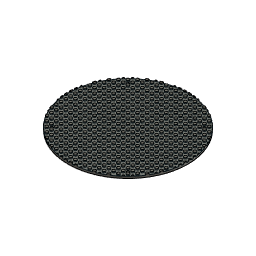
cartAssembly v25 (Autodesk Fusion 360 archive; units mm, degrees)
design "flat legosetup"
Autodesk Fusion 360 part; units mm, degrees
sketch "Sketch1" plane through (0, 0, 0) normal (0, 1, 0) x (1, 0, 0)
  line L0 (-119.9, -119.9) -> (119.9, -119.9)
  line L1 (119.9, -119.9) -> (119.9, 119.9)
  line L2 (119.9, 119.9) -> (-119.9, 119.9)
  line L3 (-119.9, 119.9) -> (-119.9, -119.9)
  line L4 (-119.9, -119.9) -> (119.9, 119.9) construction
  line L5 (119.9, -119.9) -> (-119.9, 119.9) construction
  dimension "d5" = 239.8
  dimension "d6" = 239.8
  constraint horizontal L0
  constraint perpendicular L0 L1
  constraint parallel L0 L2
  constraint parallel L1 L3
  constraint coincident L4 origin
  constraint coincident L5 origin
  measures "d5" distance of L1.end L2.end
  measures "d6" distance of L0.start L2.end
extrude "Extrude1" add sketch "Sketch1" along normal blind 3.2 makes body 1
sketch "Sketch2" plane through (0, 3.2, 0) normal (0, 1, 0) x (-1, 0, 0)
  line L0 (119.9, -119.9) -> (119.9, 119.9)
  line L1 (119.9, 119.9) -> (-119.9, 119.9)
  line L2 (-119.9, 119.9) -> (-119.9, -119.9)
  line L3 (-119.9, -119.9) -> (119.9, -119.9)
  circle A0 centre (116, -116) radius 2.4
  dimension "d9" = 4.8
  dimension "d10" = 3.9
  dimension "d11" = 3.9
  measures "d9" diameter of A0
  measures "d10" distance of L3 A0.centre
  measures "d11" distance of L0 A0.centre
extrude "Extrude2" add sketch "Sketch2" along normal blind 1.8 contours A0 bodies 1
pattern_linear "R-Pattern1" count 30 spacing 8 along (1, 0, 0) count 30 spacing 8 along (0, 0, 1) of "Extrude2"
cylinder "CylinderPrimitive1" add diameter 200 height 20 placed x (1, 0, 0) y (0, 0, -1) z (0, 1, 0) at (0, 3.2, 0) separate body makes body 2
move_body "Move1" bodies 2 to x (1, 0, 0) y (0, 1, 0) z (0, 0, 1) at (0, -10, 0)
combine "Combine1" operation intersect target body 1 tool bodies 2
sketch "Sketch4" plane through (0, 3.2, 0) normal (0, 1, 0) x (-1, 0, 0)
  arc A0 (-14.1771, 98.9899) -> (-18.2934, 98.3125) centre (0, 0) ccw
  arc A1 (-20.9263, 97.7859) -> (-18.2934, 98.3125) centre (-20, 100) ccw
  arc A2 (-20.9263, 97.7859) -> (-34.4887, 93.8644) centre (0, 0) ccw
  arc A3 (-38.3753, 92.3436) -> (-34.4887, 93.8644) centre (-36, 92) ccw
  arc A4 (-38.3753, 92.3436) -> (-41.9306, 90.7845) centre (0, 0) ccw
  arc A5 (-44.3528, 89.6261) -> (-41.9306, 90.7845) centre (-44, 92) ccw
  arc A6 (-44.3528, 89.6261) -> (-50.8497, 86.1064) centre (0, 0) ccw
  arc A7 (-54.3983, 83.9096) -> (-50.8497, 86.1064) centre (-52, 84) ccw
  arc A8 (-54.3983, 83.9096) -> (-65.673, 75.4126) centre (0, 0) ccw
  arc A9 (-67.674, 73.6222) -> (-65.673, 75.4126) centre (-68, 76) ccw
  arc A10 (-67.674, 73.6222) -> (-73.6222, 67.674) centre (0, 0) ccw
  arc A11 (-75.4126, 65.673) -> (-73.6222, 67.674) centre (-76, 68) ccw
  arc A12 (-75.4126, 65.673) -> (-83.9096, 54.3983) centre (0, 0) ccw
  arc A13 (-86.1064, 50.8497) -> (-83.9096, 54.3983) centre (-84, 52) ccw
  arc A14 (-86.1064, 50.8497) -> (-89.6261, 44.3528) centre (0, 0) ccw
  arc A15 (-90.7845, 41.9306) -> (-89.6261, 44.3528) centre (-92, 44) ccw
  arc A16 (-90.7845, 41.9306) -> (-92.3436, 38.3753) centre (0, 0) ccw
  arc A17 (-93.8644, 34.4887) -> (-92.3436, 38.3753) centre (-92, 36) ccw
  arc A18 (-93.8644, 34.4887) -> (-97.7859, 20.9263) centre (0, 0) ccw
  arc A19 (-98.3125, 18.2934) -> (-97.7859, 20.9263) centre (-100, 20) ccw
  arc A20 (-98.3125, 18.2934) -> (-98.9899, 14.1771) centre (0, 0) ccw
  arc A21 (-99.5337, 9.6457) -> (-98.9899, 14.1771) centre (-100, 12) ccw
  arc A22 (-99.5337, 9.6457) -> (-99.7955, 6.3913) centre (0, 0) ccw
  arc A23 (-99.9872, 1.6) -> (-99.7955, 6.3913) centre (-100, 4) ccw
  arc A24 (-99.9872, 1.6) -> (-99.9872, -1.6) centre (0, 0) ccw
  arc A25 (-99.7955, -6.3913) -> (-99.9872, -1.6) centre (-100, -4) ccw
  arc A26 (-99.7955, -6.3913) -> (-99.5337, -9.6457) centre (0, 0) ccw
  arc A27 (-98.9899, -14.1771) -> (-99.5337, -9.6457) centre (-100, -12) ccw
  arc A28 (-98.9899, -14.1771) -> (-98.3125, -18.2934) centre (0, 0) ccw
  arc A29 (-97.7859, -20.9263) -> (-98.3125, -18.2934) centre (-100, -20) ccw
  arc A30 (-97.7859, -20.9263) -> (-93.8644, -34.4887) centre (0, 0) ccw
  arc A31 (-92.3436, -38.3753) -> (-93.8644, -34.4887) centre (-92, -36) ccw
  arc A32 (-92.3436, -38.3753) -> (-90.7845, -41.9306) centre (0, 0) ccw
  arc A33 (-89.6261, -44.3528) -> (-90.7845, -41.9306) centre (-92, -44) ccw
  arc A34 (-89.6261, -44.3528) -> (-86.1064, -50.8497) centre (0, 0) ccw
  arc A35 (-83.9096, -54.3983) -> (-86.1064, -50.8497) centre (-84, -52) ccw
  arc A36 (-83.9096, -54.3983) -> (-75.4126, -65.673) centre (0, 0) ccw
  arc A37 (-73.6222, -67.674) -> (-75.4126, -65.673) centre (-76, -68) ccw
  arc A38 (-73.6222, -67.674) -> (-67.674, -73.6222) centre (0, 0) ccw
  arc A39 (-65.673, -75.4126) -> (-67.674, -73.6222) centre (-68, -76) ccw
  arc A40 (-65.673, -75.4126) -> (-54.3983, -83.9096) centre (0, 0) ccw
  arc A41 (-50.8497, -86.1064) -> (-54.3983, -83.9096) centre (-52, -84) ccw
  arc A42 (-50.8497, -86.1064) -> (-44.3528, -89.6261) centre (0, 0) ccw
  arc A43 (-41.9306, -90.7845) -> (-44.3528, -89.6261) centre (-44, -92) ccw
  arc A44 (-41.9306, -90.7845) -> (-38.3753, -92.3436) centre (0, 0) ccw
  arc A45 (-34.4887, -93.8644) -> (-38.3753, -92.3436) centre (-36, -92) ccw
  arc A46 (-34.4887, -93.8644) -> (-20.9263, -97.7859) centre (0, 0) ccw
  arc A47 (-18.2934, -98.3125) -> (-20.9263, -97.7859) centre (-20, -100) ccw
  arc A48 (-18.2934, -98.3125) -> (-14.1771, -98.9899) centre (0, 0) ccw
  arc A49 (-9.6457, -99.5337) -> (-14.1771, -98.9899) centre (-12, -100) ccw
  arc A50 (-9.6457, -99.5337) -> (-6.3913, -99.7955) centre (0, 0) ccw
  arc A51 (-1.6, -99.9872) -> (-6.3913, -99.7955) centre (-4, -100) ccw
  arc A52 (-1.6, -99.9872) -> (1.6, -99.9872) centre (0, 0) ccw
  arc A53 (6.3913, -99.7955) -> (1.6, -99.9872) centre (4, -100) ccw
  arc A54 (6.3913, -99.7955) -> (9.6457, -99.5337) centre (0, 0) ccw
  arc A55 (14.1771, -98.9899) -> (9.6457, -99.5337) centre (12, -100) ccw
  arc A56 (14.1771, -98.9899) -> (18.2934, -98.3125) centre (0, 0) ccw
  arc A57 (20.9263, -97.7859) -> (18.2934, -98.3125) centre (20, -100) ccw
  arc A58 (20.9263, -97.7859) -> (34.4887, -93.8644) centre (0, 0) ccw
  arc A59 (38.3753, -92.3436) -> (34.4887, -93.8644) centre (36, -92) ccw
  arc A60 (38.3753, -92.3436) -> (41.9306, -90.7845) centre (0, 0) ccw
  arc A61 (44.3528, -89.6261) -> (41.9306, -90.7845) centre (44, -92) ccw
  arc A62 (44.3528, -89.6261) -> (50.8497, -86.1064) centre (0, 0) ccw
  arc A63 (54.3983, -83.9096) -> (50.8497, -86.1064) centre (52, -84) ccw
  arc A64 (54.3983, -83.9096) -> (65.673, -75.4126) centre (0, 0) ccw
  arc A65 (67.674, -73.6222) -> (65.673, -75.4126) centre (68, -76) ccw
  arc A66 (67.674, -73.6222) -> (73.6222, -67.674) centre (0, 0) ccw
  arc A67 (75.4126, -65.673) -> (73.6222, -67.674) centre (76, -68) ccw
  arc A68 (75.4126, -65.673) -> (83.9096, -54.3983) centre (0, 0) ccw
  arc A69 (86.1064, -50.8497) -> (83.9096, -54.3983) centre (84, -52) ccw
  arc A70 (86.1064, -50.8497) -> (89.6261, -44.3528) centre (0, 0) ccw
  arc A71 (90.7845, -41.9306) -> (89.6261, -44.3528) centre (92, -44) ccw
  arc A72 (90.7845, -41.9306) -> (92.3436, -38.3753) centre (0, 0) ccw
  arc A73 (93.8644, -34.4887) -> (92.3436, -38.3753) centre (92, -36) ccw
  arc A74 (93.8644, -34.4887) -> (97.7859, -20.9263) centre (0, 0) ccw
  arc A75 (98.3125, -18.2934) -> (97.7859, -20.9263) centre (100, -20) ccw
  arc A76 (98.3125, -18.2934) -> (98.9899, -14.1771) centre (0, 0) ccw
  arc A77 (99.5337, -9.6457) -> (98.9899, -14.1771) centre (100, -12) ccw
  arc A78 (99.5337, -9.6457) -> (99.7955, -6.3913) centre (0, 0) ccw
  arc A79 (99.9872, -1.6) -> (99.7955, -6.3913) centre (100, -4) ccw
  arc A80 (99.9872, -1.6) -> (99.9872, 1.6) centre (0, 0) ccw
  arc A81 (99.7955, 6.3913) -> (99.9872, 1.6) centre (100, 4) ccw
  arc A82 (99.7955, 6.3913) -> (99.5337, 9.6457) centre (0, 0) ccw
  arc A83 (98.9899, 14.1771) -> (99.5337, 9.6457) centre (100, 12) ccw
  arc A84 (98.9899, 14.1771) -> (98.3125, 18.2934) centre (0, 0) ccw
  arc A85 (97.7859, 20.9263) -> (98.3125, 18.2934) centre (100, 20) ccw
  arc A86 (97.7859, 20.9263) -> (93.8644, 34.4887) centre (0, 0) ccw
  arc A87 (92.3436, 38.3753) -> (93.8644, 34.4887) centre (92, 36) ccw
  arc A88 (92.3436, 38.3753) -> (90.7845, 41.9306) centre (0, 0) ccw
  arc A89 (89.6261, 44.3528) -> (90.7845, 41.9306) centre (92, 44) ccw
  arc A90 (89.6261, 44.3528) -> (86.1064, 50.8497) centre (0, 0) ccw
  arc A91 (83.9096, 54.3983) -> (86.1064, 50.8497) centre (84, 52) ccw
  arc A92 (83.9096, 54.3983) -> (75.4126, 65.673) centre (0, 0) ccw
  arc A93 (73.6222, 67.674) -> (75.4126, 65.673) centre (76, 68) ccw
  arc A94 (73.6222, 67.674) -> (67.674, 73.6222) centre (0, 0) ccw
  arc A95 (65.673, 75.4126) -> (67.674, 73.6222) centre (68, 76) ccw
  arc A96 (65.673, 75.4126) -> (54.3983, 83.9096) centre (0, 0) ccw
  arc A97 (50.8497, 86.1064) -> (54.3983, 83.9096) centre (52, 84) ccw
  arc A98 (50.8497, 86.1064) -> (44.3528, 89.6261) centre (0, 0) ccw
  arc A99 (41.9306, 90.7845) -> (44.3528, 89.6261) centre (44, 92) ccw
  arc A100 (41.9306, 90.7845) -> (38.3753, 92.3436) centre (0, 0) ccw
  arc A101 (34.4887, 93.8644) -> (38.3753, 92.3436) centre (36, 92) ccw
  arc A102 (34.4887, 93.8644) -> (20.9263, 97.7859) centre (0, 0) ccw
  arc A103 (18.2934, 98.3125) -> (20.9263, 97.7859) centre (20, 100) ccw
  arc A104 (18.2934, 98.3125) -> (14.1771, 98.9899) centre (0, 0) ccw
  arc A105 (9.6457, 99.5337) -> (14.1771, 98.9899) centre (12, 100) ccw
  arc A106 (9.6457, 99.5337) -> (6.3913, 99.7955) centre (0, 0) ccw
  arc A107 (1.6, 99.9872) -> (6.3913, 99.7955) centre (4, 100) ccw
  arc A108 (1.6, 99.9872) -> (-1.6, 99.9872) centre (0, 0) ccw
  arc A109 (-6.3913, 99.7955) -> (-1.6, 99.9872) centre (-4, 100) ccw
  arc A110 (-6.3913, 99.7955) -> (-9.6457, 99.5337) centre (0, 0) ccw
  arc A111 (-14.1771, 98.9899) -> (-9.6457, 99.5337) centre (-12, 100) ccw
  circle A112 centre (-28, 92) radius 2.4
  circle A113 centre (-20, 92) radius 2.4
  circle A114 centre (-12, 92) radius 2.4
  circle A115 centre (-4, 92) radius 2.4
  circle A116 centre (4, 92) radius 2.4
  circle A117 centre (12, 92) radius 2.4
  circle A118 centre (20, 92) radius 2.4
  circle A119 centre (28, 92) radius 2.4
  circle A120 centre (-44, 84) radius 2.4
  circle A121 centre (-36, 84) radius 2.4
  circle A122 centre (-28, 84) radius 2.4
  circle A123 centre (-20, 84) radius 2.4
  circle A124 centre (-12, 84) radius 2.4
  circle A125 centre (-4, 84) radius 2.4
  circle A126 centre (4, 84) radius 2.4
  circle A127 centre (12, 84) radius 2.4
  circle A128 centre (20, 84) radius 2.4
  circle A129 centre (28, 84) radius 2.4
  circle A130 centre (36, 84) radius 2.4
  circle A131 centre (44, 84) radius 2.4
  circle A132 centre (-60, 76) radius 2.4
  circle A133 centre (-52, 76) radius 2.4
  circle A134 centre (-44, 76) radius 2.4
  circle A135 centre (-36, 76) radius 2.4
  circle A136 centre (-28, 76) radius 2.4
  circle A137 centre (-20, 76) radius 2.4
  circle A138 centre (-12, 76) radius 2.4
  circle A139 centre (-4, 76) radius 2.4
  circle A140 centre (4, 76) radius 2.4
  circle A141 centre (12, 76) radius 2.4
  circle A142 centre (20, 76) radius 2.4
  circle A143 centre (28, 76) radius 2.4
  circle A144 centre (36, 76) radius 2.4
  circle A145 centre (44, 76) radius 2.4
  circle A146 centre (52, 76) radius 2.4
  circle A147 centre (60, 76) radius 2.4
  circle A148 centre (-68, 68) radius 2.4
  circle A149 centre (-60, 68) radius 2.4
  circle A150 centre (-52, 68) radius 2.4
  circle A151 centre (-44, 68) radius 2.4
  circle A152 centre (-36, 68) radius 2.4
  circle A153 centre (-28, 68) radius 2.4
  circle A154 centre (-20, 68) radius 2.4
  circle A155 centre (-12, 68) radius 2.4
  circle A156 centre (-4, 68) radius 2.4
  circle A157 centre (4, 68) radius 2.4
  circle A158 centre (12, 68) radius 2.4
  circle A159 centre (20, 68) radius 2.4
  circle A160 centre (28, 68) radius 2.4
  circle A161 centre (36, 68) radius 2.4
  circle A162 centre (44, 68) radius 2.4
  circle A163 centre (52, 68) radius 2.4
  circle A164 centre (60, 68) radius 2.4
  circle A165 centre (68, 68) radius 2.4
  circle A166 centre (-76, 60) radius 2.4
  circle A167 centre (-68, 60) radius 2.4
  circle A168 centre (-60, 60) radius 2.4
  circle A169 centre (-52, 60) radius 2.4
  circle A170 centre (-44, 60) radius 2.4
  circle A171 centre (-36, 60) radius 2.4
  circle A172 centre (-28, 60) radius 2.4
  circle A173 centre (-20, 60) radius 2.4
  circle A174 centre (-12, 60) radius 2.4
  circle A175 centre (-4, 60) radius 2.4
  circle A176 centre (4, 60) radius 2.4
  circle A177 centre (12, 60) radius 2.4
  circle A178 centre (20, 60) radius 2.4
  circle A179 centre (28, 60) radius 2.4
  circle A180 centre (36, 60) radius 2.4
  circle A181 centre (44, 60) radius 2.4
  circle A182 centre (52, 60) radius 2.4
  circle A183 centre (60, 60) radius 2.4
  circle A184 centre (68, 60) radius 2.4
  circle A185 centre (76, 60) radius 2.4
  circle A186 centre (-76, 52) radius 2.4
  circle A187 centre (-68, 52) radius 2.4
  circle A188 centre (-60, 52) radius 2.4
  circle A189 centre (-52, 52) radius 2.4
  circle A190 centre (-44, 52) radius 2.4
  circle A191 centre (-36, 52) radius 2.4
  circle A192 centre (-28, 52) radius 2.4
  circle A193 centre (-20, 52) radius 2.4
  circle A194 centre (-12, 52) radius 2.4
  circle A195 centre (-4, 52) radius 2.4
  circle A196 centre (4, 52) radius 2.4
  circle A197 centre (12, 52) radius 2.4
  circle A198 centre (20, 52) radius 2.4
  circle A199 centre (28, 52) radius 2.4
  circle A200 centre (36, 52) radius 2.4
  circle A201 centre (44, 52) radius 2.4
  circle A202 centre (52, 52) radius 2.4
  circle A203 centre (60, 52) radius 2.4
  circle A204 centre (68, 52) radius 2.4
  circle A205 centre (76, 52) radius 2.4
  circle A206 centre (-84, 44) radius 2.4
  circle A207 centre (-76, 44) radius 2.4
  circle A208 centre (-68, 44) radius 2.4
  circle A209 centre (-60, 44) radius 2.4
  circle A210 centre (-52, 44) radius 2.4
  circle A211 centre (-44, 44) radius 2.4
  circle A212 centre (-36, 44) radius 2.4
  circle A213 centre (-28, 44) radius 2.4
  circle A214 centre (-20, 44) radius 2.4
  circle A215 centre (-12, 44) radius 2.4
  circle A216 centre (-4, 44) radius 2.4
  circle A217 centre (4, 44) radius 2.4
  circle A218 centre (12, 44) radius 2.4
  circle A219 centre (20, 44) radius 2.4
  circle A220 centre (28, 44) radius 2.4
  circle A221 centre (36, 44) radius 2.4
  circle A222 centre (44, 44) radius 2.4
  circle A223 centre (52, 44) radius 2.4
  circle A224 centre (60, 44) radius 2.4
  circle A225 centre (68, 44) radius 2.4
  circle A226 centre (76, 44) radius 2.4
  circle A227 centre (84, 44) radius 2.4
  circle A228 centre (-84, 36) radius 2.4
  circle A229 centre (-76, 36) radius 2.4
  circle A230 centre (-68, 36) radius 2.4
  circle A231 centre (-60, 36) radius 2.4
  circle A232 centre (-52, 36) radius 2.4
  circle A233 centre (-44, 36) radius 2.4
  circle A234 centre (-36, 36) radius 2.4
  circle A235 centre (-28, 36) radius 2.4
  circle A236 centre (-20, 36) radius 2.4
  circle A237 centre (-12, 36) radius 2.4
  circle A238 centre (-4, 36) radius 2.4
  circle A239 centre (4, 36) radius 2.4
  circle A240 centre (12, 36) radius 2.4
  circle A241 centre (20, 36) radius 2.4
  circle A242 centre (28, 36) radius 2.4
  circle A243 centre (36, 36) radius 2.4
  circle A244 centre (44, 36) radius 2.4
  circle A245 centre (52, 36) radius 2.4
  circle A246 centre (60, 36) radius 2.4
  circle A247 centre (68, 36) radius 2.4
  circle A248 centre (76, 36) radius 2.4
  circle A249 centre (84, 36) radius 2.4
  circle A250 centre (-92, 28) radius 2.4
  circle A251 centre (-84, 28) radius 2.4
  circle A252 centre (-76, 28) radius 2.4
  circle A253 centre (-68, 28) radius 2.4
  circle A254 centre (-60, 28) radius 2.4
  circle A255 centre (-52, 28) radius 2.4
  circle A256 centre (-44, 28) radius 2.4
  circle A257 centre (-36, 28) radius 2.4
  circle A258 centre (-28, 28) radius 2.4
  circle A259 centre (-20, 28) radius 2.4
  circle A260 centre (-12, 28) radius 2.4
  circle A261 centre (-4, 28) radius 2.4
  circle A262 centre (4, 28) radius 2.4
  circle A263 centre (12, 28) radius 2.4
  circle A264 centre (20, 28) radius 2.4
  circle A265 centre (28, 28) radius 2.4
  circle A266 centre (36, 28) radius 2.4
  circle A267 centre (44, 28) radius 2.4
  circle A268 centre (52, 28) radius 2.4
  circle A269 centre (60, 28) radius 2.4
  circle A270 centre (68, 28) radius 2.4
  circle A271 centre (76, 28) radius 2.4
  circle A272 centre (84, 28) radius 2.4
  circle A273 centre (92, 28) radius 2.4
  circle A274 centre (-92, 20) radius 2.4
  circle A275 centre (-84, 20) radius 2.4
  circle A276 centre (-76, 20) radius 2.4
  circle A277 centre (-68, 20) radius 2.4
  circle A278 centre (-60, 20) radius 2.4
  circle A279 centre (-52, 20) radius 2.4
  circle A280 centre (-44, 20) radius 2.4
  circle A281 centre (-36, 20) radius 2.4
  circle A282 centre (-28, 20) radius 2.4
  circle A283 centre (-20, 20) radius 2.4
  circle A284 centre (-12, 20) radius 2.4
  circle A285 centre (-4, 20) radius 2.4
  circle A286 centre (4, 20) radius 2.4
  circle A287 centre (12, 20) radius 2.4
  circle A288 centre (20, 20) radius 2.4
  circle A289 centre (28, 20) radius 2.4
  circle A290 centre (36, 20) radius 2.4
  circle A291 centre (44, 20) radius 2.4
  circle A292 centre (52, 20) radius 2.4
  circle A293 centre (60, 20) radius 2.4
  circle A294 centre (68, 20) radius 2.4
  circle A295 centre (76, 20) radius 2.4
  circle A296 centre (84, 20) radius 2.4
  circle A297 centre (92, 20) radius 2.4
  circle A298 centre (-92, 12) radius 2.4
  circle A299 centre (-84, 12) radius 2.4
  circle A300 centre (-76, 12) radius 2.4
  circle A301 centre (-68, 12) radius 2.4
  circle A302 centre (-60, 12) radius 2.4
  circle A303 centre (-52, 12) radius 2.4
  circle A304 centre (-44, 12) radius 2.4
  circle A305 centre (-36, 12) radius 2.4
  circle A306 centre (-28, 12) radius 2.4
  circle A307 centre (-20, 12) radius 2.4
  circle A308 centre (-12, 12) radius 2.4
  circle A309 centre (-4, 12) radius 2.4
  circle A310 centre (4, 12) radius 2.4
  circle A311 centre (12, 12) radius 2.4
  circle A312 centre (20, 12) radius 2.4
  circle A313 centre (28, 12) radius 2.4
  circle A314 centre (36, 12) radius 2.4
  circle A315 centre (44, 12) radius 2.4
  circle A316 centre (52, 12) radius 2.4
  circle A317 centre (60, 12) radius 2.4
  circle A318 centre (68, 12) radius 2.4
  circle A319 centre (76, 12) radius 2.4
  circle A320 centre (84, 12) radius 2.4
  circle A321 centre (92, 12) radius 2.4
  circle A322 centre (-92, 4) radius 2.4
  circle A323 centre (-84, 4) radius 2.4
  circle A324 centre (-76, 4) radius 2.4
  circle A325 centre (-68, 4) radius 2.4
  circle A326 centre (-60, 4) radius 2.4
  circle A327 centre (-52, 4) radius 2.4
  circle A328 centre (-44, 4) radius 2.4
  circle A329 centre (-36, 4) radius 2.4
  circle A330 centre (-28, 4) radius 2.4
  circle A331 centre (-20, 4) radius 2.4
  circle A332 centre (-12, 4) radius 2.4
  circle A333 centre (-4, 4) radius 2.4
  circle A334 centre (4, 4) radius 2.4
  circle A335 centre (12, 4) radius 2.4
  circle A336 centre (20, 4) radius 2.4
  circle A337 centre (28, 4) radius 2.4
  circle A338 centre (36, 4) radius 2.4
  circle A339 centre (44, 4) radius 2.4
  circle A340 centre (52, 4) radius 2.4
  circle A341 centre (60, 4) radius 2.4
  circle A342 centre (68, 4) radius 2.4
  circle A343 centre (76, 4) radius 2.4
  circle A344 centre (84, 4) radius 2.4
  circle A345 centre (92, 4) radius 2.4
  circle A346 centre (-92, -4) radius 2.4
  circle A347 centre (-84, -4) radius 2.4
  circle A348 centre (-76, -4) radius 2.4
  circle A349 centre (-68, -4) radius 2.4
  circle A350 centre (-60, -4) radius 2.4
  circle A351 centre (-52, -4) radius 2.4
  circle A352 centre (-44, -4) radius 2.4
  circle A353 centre (-36, -4) radius 2.4
  circle A354 centre (-28, -4) radius 2.4
  circle A355 centre (-20, -4) radius 2.4
  circle A356 centre (-12, -4) radius 2.4
  circle A357 centre (-4, -4) radius 2.4
  circle A358 centre (4, -4) radius 2.4
  circle A359 centre (12, -4) radius 2.4
  circle A360 centre (20, -4) radius 2.4
  circle A361 centre (28, -4) radius 2.4
  circle A362 centre (36, -4) radius 2.4
  circle A363 centre (44, -4) radius 2.4
  circle A364 centre (52, -4) radius 2.4
  circle A365 centre (60, -4) radius 2.4
  circle A366 centre (68, -4) radius 2.4
  circle A367 centre (76, -4) radius 2.4
  circle A368 centre (84, -4) radius 2.4
  circle A369 centre (92, -4) radius 2.4
  circle A370 centre (-92, -12) radius 2.4
  circle A371 centre (-84, -12) radius 2.4
  circle A372 centre (-76, -12) radius 2.4
  circle A373 centre (-68, -12) radius 2.4
  circle A374 centre (-60, -12) radius 2.4
  circle A375 centre (-52, -12) radius 2.4
  circle A376 centre (-44, -12) radius 2.4
  circle A377 centre (-36, -12) radius 2.4
  circle A378 centre (-28, -12) radius 2.4
  circle A379 centre (-20, -12) radius 2.4
  circle A380 centre (-12, -12) radius 2.4
  circle A381 centre (-4, -12) radius 2.4
  circle A382 centre (4, -12) radius 2.4
  circle A383 centre (12, -12) radius 2.4
  circle A384 centre (20, -12) radius 2.4
  circle A385 centre (28, -12) radius 2.4
  circle A386 centre (36, -12) radius 2.4
  circle A387 centre (44, -12) radius 2.4
  circle A388 centre (52, -12) radius 2.4
  circle A389 centre (60, -12) radius 2.4
  circle A390 centre (68, -12) radius 2.4
  circle A391 centre (76, -12) radius 2.4
  circle A392 centre (84, -12) radius 2.4
  circle A393 centre (92, -12) radius 2.4
  circle A394 centre (-92, -20) radius 2.4
  circle A395 centre (-84, -20) radius 2.4
  circle A396 centre (-76, -20) radius 2.4
  circle A397 centre (-68, -20) radius 2.4
  circle A398 centre (-60, -20) radius 2.4
  circle A399 centre (-52, -20) radius 2.4
  circle A400 centre (-44, -20) radius 2.4
  circle A401 centre (-36, -20) radius 2.4
  circle A402 centre (-28, -20) radius 2.4
  circle A403 centre (-20, -20) radius 2.4
  circle A404 centre (-12, -20) radius 2.4
  circle A405 centre (-4, -20) radius 2.4
  circle A406 centre (4, -20) radius 2.4
  circle A407 centre (12, -20) radius 2.4
  circle A408 centre (20, -20) radius 2.4
  circle A409 centre (28, -20) radius 2.4
  circle A410 centre (36, -20) radius 2.4
  circle A411 centre (44, -20) radius 2.4
  circle A412 centre (52, -20) radius 2.4
  circle A413 centre (60, -20) radius 2.4
  circle A414 centre (68, -20) radius 2.4
  circle A415 centre (76, -20) radius 2.4
  circle A416 centre (84, -20) radius 2.4
  circle A417 centre (92, -20) radius 2.4
  circle A418 centre (-92, -28) radius 2.4
  circle A419 centre (-84, -28) radius 2.4
  circle A420 centre (-76, -28) radius 2.4
  circle A421 centre (-68, -28) radius 2.4
  circle A422 centre (-60, -28) radius 2.4
  circle A423 centre (-52, -28) radius 2.4
  circle A424 centre (-44, -28) radius 2.4
  circle A425 centre (-36, -28) radius 2.4
  circle A426 centre (-28, -28) radius 2.4
  circle A427 centre (-20, -28) radius 2.4
  circle A428 centre (-12, -28) radius 2.4
  circle A429 centre (-4, -28) radius 2.4
  circle A430 centre (4, -28) radius 2.4
  circle A431 centre (12, -28) radius 2.4
  circle A432 centre (20, -28) radius 2.4
  circle A433 centre (28, -28) radius 2.4
  circle A434 centre (36, -28) radius 2.4
  circle A435 centre (44, -28) radius 2.4
  circle A436 centre (52, -28) radius 2.4
  circle A437 centre (60, -28) radius 2.4
  circle A438 centre (68, -28) radius 2.4
  circle A439 centre (76, -28) radius 2.4
  circle A440 centre (84, -28) radius 2.4
  circle A441 centre (92, -28) radius 2.4
  circle A442 centre (-84, -36) radius 2.4
  circle A443 centre (-76, -36) radius 2.4
  circle A444 centre (-68, -36) radius 2.4
  circle A445 centre (-60, -36) radius 2.4
  circle A446 centre (-52, -36) radius 2.4
  circle A447 centre (-44, -36) radius 2.4
  circle A448 centre (-36, -36) radius 2.4
  circle A449 centre (-28, -36) radius 2.4
  circle A450 centre (-20, -36) radius 2.4
  circle A451 centre (-12, -36) radius 2.4
  circle A452 centre (-4, -36) radius 2.4
  circle A453 centre (4, -36) radius 2.4
  circle A454 centre (12, -36) radius 2.4
  circle A455 centre (20, -36) radius 2.4
  circle A456 centre (28, -36) radius 2.4
  circle A457 centre (36, -36) radius 2.4
  circle A458 centre (44, -36) radius 2.4
  circle A459 centre (52, -36) radius 2.4
  circle A460 centre (60, -36) radius 2.4
  circle A461 centre (68, -36) radius 2.4
  circle A462 centre (76, -36) radius 2.4
  circle A463 centre (84, -36) radius 2.4
  circle A464 centre (-84, -44) radius 2.4
  circle A465 centre (-76, -44) radius 2.4
  circle A466 centre (-68, -44) radius 2.4
  circle A467 centre (-60, -44) radius 2.4
  circle A468 centre (-52, -44) radius 2.4
  circle A469 centre (-44, -44) radius 2.4
  circle A470 centre (-36, -44) radius 2.4
  circle A471 centre (-28, -44) radius 2.4
  circle A472 centre (-20, -44) radius 2.4
  circle A473 centre (-12, -44) radius 2.4
  circle A474 centre (-4, -44) radius 2.4
  circle A475 centre (4, -44) radius 2.4
  circle A476 centre (12, -44) radius 2.4
  circle A477 centre (20, -44) radius 2.4
  circle A478 centre (28, -44) radius 2.4
  circle A479 centre (36, -44) radius 2.4
  circle A480 centre (44, -44) radius 2.4
  circle A481 centre (52, -44) radius 2.4
  circle A482 centre (60, -44) radius 2.4
  circle A483 centre (68, -44) radius 2.4
  circle A484 centre (76, -44) radius 2.4
  circle A485 centre (84, -44) radius 2.4
  circle A486 centre (-76, -52) radius 2.4
  circle A487 centre (-68, -52) radius 2.4
  circle A488 centre (-60, -52) radius 2.4
  circle A489 centre (-52, -52) radius 2.4
  circle A490 centre (-44, -52) radius 2.4
  circle A491 centre (-36, -52) radius 2.4
  circle A492 centre (-28, -52) radius 2.4
  circle A493 centre (-20, -52) radius 2.4
  circle A494 centre (-12, -52) radius 2.4
  circle A495 centre (-4, -52) radius 2.4
  circle A496 centre (4, -52) radius 2.4
  circle A497 centre (12, -52) radius 2.4
  circle A498 centre (20, -52) radius 2.4
  circle A499 centre (28, -52) radius 2.4
  circle A500 centre (36, -52) radius 2.4
  circle A501 centre (44, -52) radius 2.4
  circle A502 centre (52, -52) radius 2.4
  circle A503 centre (60, -52) radius 2.4
  circle A504 centre (68, -52) radius 2.4
  circle A505 centre (76, -52) radius 2.4
  circle A506 centre (-76, -60) radius 2.4
  circle A507 centre (-68, -60) radius 2.4
  circle A508 centre (-60, -60) radius 2.4
  circle A509 centre (-52, -60) radius 2.4
  circle A510 centre (-44, -60) radius 2.4
  circle A511 centre (-36, -60) radius 2.4
  circle A512 centre (-28, -60) radius 2.4
  circle A513 centre (-20, -60) radius 2.4
  circle A514 centre (-12, -60) radius 2.4
  circle A515 centre (-4, -60) radius 2.4
  circle A516 centre (4, -60) radius 2.4
  circle A517 centre (12, -60) radius 2.4
  circle A518 centre (20, -60) radius 2.4
  circle A519 centre (28, -60) radius 2.4
  circle A520 centre (36, -60) radius 2.4
  circle A521 centre (44, -60) radius 2.4
  circle A522 centre (52, -60) radius 2.4
  circle A523 centre (60, -60) radius 2.4
  circle A524 centre (68, -60) radius 2.4
  circle A525 centre (76, -60) radius 2.4
  circle A526 centre (-68, -68) radius 2.4
  circle A527 centre (-60, -68) radius 2.4
  circle A528 centre (-52, -68) radius 2.4
  circle A529 centre (-44, -68) radius 2.4
  circle A530 centre (-36, -68) radius 2.4
  circle A531 centre (-28, -68) radius 2.4
  circle A532 centre (-20, -68) radius 2.4
  circle A533 centre (-12, -68) radius 2.4
  circle A534 centre (-4, -68) radius 2.4
  circle A535 centre (4, -68) radius 2.4
  circle A536 centre (12, -68) radius 2.4
  circle A537 centre (20, -68) radius 2.4
  circle A538 centre (28, -68) radius 2.4
  circle A539 centre (36, -68) radius 2.4
  circle A540 centre (44, -68) radius 2.4
  circle A541 centre (52, -68) radius 2.4
  circle A542 centre (60, -68) radius 2.4
  circle A543 centre (68, -68) radius 2.4
  circle A544 centre (-60, -76) radius 2.4
  circle A545 centre (-52, -76) radius 2.4
  circle A546 centre (-44, -76) radius 2.4
  circle A547 centre (-36, -76) radius 2.4
  circle A548 centre (-28, -76) radius 2.4
  circle A549 centre (-20, -76) radius 2.4
  circle A550 centre (-12, -76) radius 2.4
  circle A551 centre (-4, -76) radius 2.4
  circle A552 centre (4, -76) radius 2.4
  circle A553 centre (12, -76) radius 2.4
  circle A554 centre (20, -76) radius 2.4
  circle A555 centre (28, -76) radius 2.4
  circle A556 centre (36, -76) radius 2.4
  circle A557 centre (44, -76) radius 2.4
  circle A558 centre (52, -76) radius 2.4
  circle A559 centre (60, -76) radius 2.4
  circle A560 centre (-44, -84) radius 2.4
  circle A561 centre (-36, -84) radius 2.4
  circle A562 centre (-28, -84) radius 2.4
  circle A563 centre (-20, -84) radius 2.4
  circle A564 centre (-12, -84) radius 2.4
  circle A565 centre (-4, -84) radius 2.4
  circle A566 centre (4, -84) radius 2.4
  circle A567 centre (12, -84) radius 2.4
  circle A568 centre (20, -84) radius 2.4
  circle A569 centre (28, -84) radius 2.4
  circle A570 centre (36, -84) radius 2.4
  circle A571 centre (44, -84) radius 2.4
  circle A572 centre (-28, -92) radius 2.4
  circle A573 centre (-20, -92) radius 2.4
  circle A574 centre (-12, -92) radius 2.4
  circle A575 centre (-4, -92) radius 2.4
  circle A576 centre (4, -92) radius 2.4
  circle A577 centre (12, -92) radius 2.4
  circle A578 centre (20, -92) radius 2.4
  circle A579 centre (28, -92) radius 2.4
cylinder "CylinderPrimitive2" cut diameter 4 height -10 placed x (1, 0, 0) y (0, 0, -1) z (0, 1, 0) at (-64.0864, 3.2, 63.542) bodies 1
cylinder "CylinderPrimitive3" cut diameter 4 height -10 placed x (1, 0, 0) y (0, 0, -1) z (0, 1, 0) at (63.9501, 3.2, 63.7574) bodies 1
cylinder "CylinderPrimitive4" cut diameter 4 height -5 placed x (1, 0, 0) y (0, 0, -1) z (0, 1, 0) at (-63.9523, 3.2, -63.9679) bodies 1
cylinder "CylinderPrimitive5" cut diameter 4 height -5 placed x (1, 0, 0) y (0, 0, -1) z (0, 1, 0) at (63.9795, 3.2, -63.8207) bodies 1
equation "LENGTH = 30"
equation "WIDTH = 30"
equation "HIGH = LOW"
equation "LOW = 3.2 mm"
equation "d5 = ( LENGTH * 8 mm ) - 0.2 mm"
equation "d6 = ( WIDTH * 8 mm ) - 0.2 mm"
equation "d7 = HIGH"
equation "d14 = LENGTH"
equation "d15 = WIDTH"
